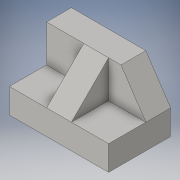
# Autodesk Inventor part: Figure 7_28_4
Saved by Autodesk Inventor 2016 (Build 200138000, 138)
## iProperties
Created: 2016-07-19
Part Number: Figure 7_28_4
Material: Generic
Document SubType Name: Modeling
Designer: cfkguest
Density: 1 g/cm^3
Appearance: Default
Author: cfkguest
Autodesk Inventor part; units mm, degrees
ref_plane "YZ Plane" through (0, 0, 0) normal (1, 0, 0) x (0, 1, 0)
ref_plane "XZ Plane" through (0, 0, 0) normal (0, 1, 0) x (-1, 0, 0)
ref_plane "XY Plane" through (0, 0, 0) normal (0, 0, 1) x (1, 0, 0)
sketch "Sketch1" plane through (0, 0, 0) normal (0, 0, 1) x (1, 0, 0)
  line L0 (-19.5098, 12.246) -> (31.2902, 12.246)
  line L1 (31.2902, 12.246) -> (31.2902, -19.504)
  line L2 (31.2902, -19.504) -> (-19.5098, -19.504)
  line L3 (-19.5098, -19.504) -> (-19.5098, 12.246)
  point P0 (0, 0)
  dimension "d0" = 50.8
  dimension "d1" = 31.75
  constraints: 8 end point, 2 parallel, 1 horizontal, 1 perpendicular
  measures "d0" distance of L0.start L0.end
  measures "d1" distance of L0.end L1.end
extrude "Extrusion1" add sketch "Sketch1" along normal blind 31.75
sketch "Sketch2" plane through (0, 0, 31.75) normal (0, 0, 1) x (1, 0, 0)
  line L0 (31.2902, 12.246) -> (-19.5098, 12.246) projected
  line L1 (-19.5098, 12.246) -> (-0.4598, 12.246)
  line L2 (-0.4598, 12.246) -> (-0.4598, -6.804)
  line L3 (-0.4598, -6.804) -> (-19.5098, -6.804)
  line L4 (-19.5098, -6.804) -> (-19.5098, 12.246)
  line L5 (31.2902, 12.246) -> (12.2402, 12.246)
  line L6 (12.2402, 12.246) -> (12.2402, -6.804)
  line L7 (12.2402, -6.804) -> (31.2902, -6.804)
  line L8 (31.2902, -6.804) -> (31.2902, 12.246)
  line L9 (31.2902, -19.504) -> (-19.5098, -19.504) projected
  point P0 (0, 0)
  dimension "d4" = 12.7
  dimension "d5" = 12.7
  dimension "d6" = 19.05
  dimension "d7" = 19.05
  constraints: 16 end point, 4 parallel, 2 horizontal, 2 perpendicular
  measures "d4" distance between parallel lines of L9 L3
  measures "d5" distance between parallel lines of L9 L7
  measures "d6" distance between parallel lines of L8 L6
  measures "d7" distance between parallel lines of L2 L4
extrude "Extrusion2" cut sketch "Sketch2" against normal blind 19.05
sketch "Sketch3" plane through (12.2402, -6.804, 31.75) normal (1, 0, 0) x (0, 0, -1)
  line L0 (0, 0) -> (19.05, 0) projected
  line L1 (19.05, 0) -> (19.05, 19.05) projected
  line L2 (0, 0) -> (19.05, 19.05)
  line L3 (0, 19.05) -> (19.05, 19.05) projected
  line L4 (19.05, 19.05) -> (0, 19.05)
  line L5 (0, 0) -> (0, 19.05) projected
  line L6 (0, 19.05) -> (0, 0)
  point P0 (31.75, 6.804)
  constraints: 6 end point, 1 collinear, 1 perpendicular
extrude "Extrusion3" cut sketch "Sketch3" against normal blind 19.05 contours L5 L3 L2
sketch "Sketch4" plane through (0, 0, 12.7) normal (0, 0, 1) x (1, 0, 0)
  line L0 (31.2902, -19.504) -> (31.2902, -6.804) projected
  line L1 (31.2902, -6.804) -> (18.5902, 12.246)
  line L2 (12.2402, 12.246) -> (31.2902, 12.246) projected
  line L3 (18.5902, 12.246) -> (31.2902, 12.246)
  line L4 (31.2902, 12.246) -> (31.2902, -6.804)
  point P0 (0, 0)
  dimension "d12" = 6.35
  constraints: 6 end point, 1 horizontal, 1 perpendicular, 1 point on line
  measures "d12" distance of L2.start L1.end
extrude "Extrusion4" cut sketch "Sketch4" against normal blind 19.05
body "Solid1"
